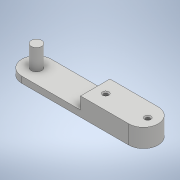
# Autodesk Inventor part: элемент-1
Saved by Autodesk Inventor 2020 (Build 240168000, 168)
## iProperties
Created: 2020-01-23
Part Number: элемент-1
Material: Типовые
Document SubType Name: Modeling
Designer: Css38
Density: 1 g/cm^3
Appearance: По умолчанию
Author: Css38
Autodesk Inventor part; units mm, degrees
ref_plane "YZ Plane" through (0, 0, 0) normal (1, 0, 0) x (0, 1, 0)
ref_plane "XZ Plane" through (0, 0, 0) normal (0, 1, 0) x (-1, 0, 0)
ref_plane "XY Plane" through (0, 0, 0) normal (0, 0, 1) x (1, 0, 0)
sketch "Эскиз1" plane through (0, 0, 0) normal (0, 0, 1) x (1, 0, 0)
  line L0 (0, 0) -> (25.5, 0) construction
  line L1 (0, -3.5) -> (25.5, -3.5)
  line L2 (25.5, 3.5) -> (0, 3.5)
  arc A0 (0, 3.5) -> (0, -3.5) centre (0, 0) ccw
  arc A1 (25.5, -3.5) -> (25.5, 3.5) centre (25.5, 0) ccw
  point P0 (12.75, 0)
  dimension "d3" = 25.5
  dimension "d4" = 7
  constraints: 8 end point, 4 point on circle, 4 tangent, 2 centre point, 1 horizontal, 1 midpoint, 1 parallel
  measures "d3" distance of L0.start L0.end
  measures "d4" diameter of A1
extrude "Выдавливание1" add sketch "Эскиз1" along normal blind 1.5
sketch "Эскиз2" plane through (0, 0, 1.5) normal (0, 0, 1) x (1, 0, 0)
  circle A0 centre (0, 0) radius 1.25
  dimension "d7" = 2.5
  constraints: 1 centre point, 1 coincident
  measures "d7" diameter of A0
extrude "Выдавливание2" add sketch "Эскиз2" along normal blind 5
sketch "Эскиз4" plane through (0, 0, 1.5) normal (0, 0, 1) x (1, 0, 0)
  line L0 (0, -3.5) -> (25.5, -3.5) construction
  arc A0 (0, 3.5) -> (0, -3.5) centre (0, 0) ccw construction
  line L1 (25.5, 3.5) -> (0, 3.5) construction
  arc A1 (25.5, -3.5) -> (25.5, 3.5) centre (25.5, 0) ccw construction
  line L2 (25.5, -3.5) -> (14, -3.5)
  line L3 (14, 3.5) -> (25.5, 3.5)
  arc A2 (25.5, -3.5) -> (25.5, 3.5) centre (25.5, 0) ccw
  line L4 (14, 3.5) -> (14, -3.5)
  dimension "d15" = 11.5
  constraints: 6 end point, 2 parallel, 2 point on circle, 2 tangent, 1 centre point, 1 coincident, 1 concentric, 1 horizontal
  measures "d15" distance of L2.start L2.end
extrude "Выдавливание4" add sketch "Эскиз4" along normal blind 2.9
sketch "Эскиз5" plane through (0, 0, 4.4) normal (0, 0, 1) x (1, 0, 0)
  circle A0 centre (26.5, 0) radius 0.5
  circle A1 centre (16.5, 0) radius 0.5
  line L0 (16.5, 0) -> (21.5, 0) construction
  line L1 (21.5, 0) -> (26.5, 0) construction
  arc A2 (25.5, -3.5) -> (25.5, 3.5) centre (25.5, 0) ccw construction
  point P0 (0, 0)
  point P1 (29, 0)
  dimension "d18" = 1
  dimension "d25" = 10
  dimension "d26" = 2.5
  constraints: 4 end point, 2 centre point, 2 collinear, 2 horizontal alignment, 1 equal radius, 1 horizontal, 1 point on circle
  measures "d18" diameter of A0
  measures "d25" distance of L0.start L1.end
  measures "d26" distance of point (29, 0) L1.end
hole "Отверстие1" at (16.5, 0, 4.4) at (26.5, 0, 4.4) direction (0, 0, -1) diameter 1 end through all countersink diameter 1.5 countersink angle 90
